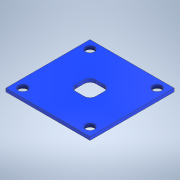
# Autodesk Inventor part: arena_middle
Saved by Autodesk Inventor 2021 (Build 250183000, 183)
## iProperties
Created: 2021-02-15
Part Number: arena_middle
Material: Generic
Document SubType Name: Modeling
Designer: lobato
Density: 1 g/cm^3
Appearance: Default
Author: lobato
Autodesk Inventor part; units mm, degrees
ref_plane "YZ Plane" through (0, 0, 0) normal (1, 0, 0) x (0, 1, 0)
ref_plane "XZ Plane" through (0, 0, 0) normal (0, 1, 0) x (-1, 0, 0)
ref_plane "XY Plane" through (0, 0, 0) normal (0, 0, 1) x (1, 0, 0)
sketch "Sketch1" plane through (0, 0, 0) normal (0, 1, 0) x (-1, 0, 0)
  line L0 (25, 25) -> (-25, 25)
  line L1 (-25, 25) -> (-25, -25)
  line L2 (-25, -25) -> (25, -25)
  line L3 (25, -25) -> (25, 25)
  line L4 (25, 25) -> (-25, -25) construction
  line L5 (-25, 25) -> (25, -25) construction
  line L6 (6, 6) -> (-6, 6)
  line L7 (-6, 6) -> (-6, -6)
  line L8 (-6, -6) -> (6, -6)
  line L9 (6, -6) -> (6, 6)
  line L10 (6, 6) -> (-6, -6) construction
  line L11 (-6, 6) -> (6, -6) construction
  line L12 (20, 20) -> (-20, 20) construction
  line L13 (-20, 20) -> (-20, -20) construction
  line L14 (-20, -20) -> (20, -20) construction
  line L15 (20, -20) -> (20, 20) construction
  line L16 (20, 20) -> (-20, -20) construction
  line L17 (-20, 20) -> (20, -20) construction
  circle A0 centre (20, 20) radius 2.625
  circle A1 centre (20, -20) radius 2.625
  circle A2 centre (-20, -20) radius 2.625
  circle A3 centre (-20, 20) radius 2.625
  point P0 (0, 0)
  dimension "d0" = 50
  dimension "d1" = 50
  dimension "d2" = 12
  dimension "d3" = 12
  dimension "d4" = 40
  dimension "d5" = 40
  dimension "d6" = 5.25
  dimension "d7" = 5.25
  dimension "d8" = 5.25
  dimension "d9" = 5.25
  constraints: 36 end point, 6 midpoint, 6 parallel, 4 centre point, 4 coincident, 3 horizontal, 3 perpendicular
  measures "d0" distance of L2.end L1.end
  measures "d1" distance of L1.end L0.end
  measures "d2" distance of L8.end L7.end
  measures "d3" distance of L7.end L6.end
  measures "d4" distance of L14.end L13.end
  measures "d5" distance of L13.end L12.end
  measures "d6" diameter of A0
  measures "d7" diameter of A1
  measures "d8" diameter of A2
  measures "d9" diameter of A3
extrude "Extrusion1" add sketch "Sketch1" along normal blind 2
fillet "Fillet1" radius 3.5 4 edges at (-6, 1, 6) (-6, 1, -6) (6, 1, -6) (6, 1, 6)
body "Solid1"
